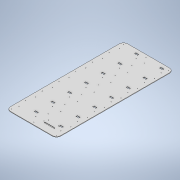
# Autodesk Inventor part: back_Box
Saved by Autodesk Inventor 2020 (Build 240168000, 168)
## iProperties
Created: 2020-07-08
Part Number: back_Box
Material: Generic
Document SubType Name: Modeling
Designer: gerac
Density: 1 g/cm^3
Appearance: Default
Author: gerac
Autodesk Inventor part; units mm, degrees
ref_plane "YZ Plane" through (0, 0, 0) normal (1, 0, 0) x (0, 1, 0)
ref_plane "XZ Plane" through (0, 0, 0) normal (0, 1, 0) x (-1, 0, 0)
ref_plane "XY Plane" through (0, 0, 0) normal (0, 0, 1) x (1, 0, 0)
sketch "Sketch1" plane through (0, 0, 0) normal (0, 1, 0) x (-1, 0, 0)
  line L0 (144, 336) -> (-144, 336)
  line L1 (-144, 336) -> (-144, -336)
  line L2 (-144, -336) -> (144, -336)
  line L3 (144, -336) -> (144, 336)
  line L4 (144, 336) -> (-144, -336) construction
  line L5 (-144, 336) -> (144, -336) construction
  circle A0 centre (-24, 288) radius 1.25
  circle A1 centre (-121, 288) radius 1.25
  circle A2 centre (-24, 192) radius 1.25
  circle A3 centre (-121, 192) radius 1.25
  circle A4 centre (-24, 96) radius 1.25
  circle A5 centre (-121, 96) radius 1.25
  circle A6 centre (-24, 0) radius 1.25
  circle A7 centre (-121, 0) radius 1.25
  circle A8 centre (-24, -96) radius 1.25
  circle A9 centre (-121, -96) radius 1.25
  circle A10 centre (-24, -192) radius 1.25
  circle A11 centre (-121, -192) radius 1.25
  circle A12 centre (-24, -288) radius 1.25
  circle A13 centre (-121, -288) radius 1.25
  circle A14 centre (120, 288) radius 1.25
  circle A15 centre (23, 288) radius 1.25
  circle A16 centre (120, 192) radius 1.25
  circle A17 centre (23, 192) radius 1.25
  circle A18 centre (120, 96) radius 1.25
  circle A19 centre (23, 96) radius 1.25
  circle A20 centre (120, 0) radius 1.25
  circle A21 centre (23, 0) radius 1.25
  circle A22 centre (120, -96) radius 1.25
  circle A23 centre (23, -96) radius 1.25
  circle A24 centre (120, -192) radius 1.25
  circle A25 centre (23, -192) radius 1.25
  circle A26 centre (120, -288) radius 1.25
  circle A27 centre (23, -288) radius 1.25
  line L6 (-92.1, 269) -> (-109.1, 269)
  line L7 (-109.1, 269) -> (-109.1, 261)
  line L8 (-109.1, 261) -> (-92.1, 261)
  line L9 (-92.1, 261) -> (-92.1, 269)
  line L10 (-92.1, 269) -> (-109.1, 261) construction
  line L11 (-109.1, 269) -> (-92.1, 261) construction
  line L12 (-92.1, 165) -> (-92.1, 173)
  line L13 (-92.1, 173) -> (-109.1, 173)
  line L14 (-109.1, 173) -> (-109.1, 165)
  line L15 (-109.1, 165) -> (-92.1, 165)
  line L16 (-92.1, 69) -> (-92.1, 77)
  line L17 (-92.1, 77) -> (-109.1, 77)
  line L18 (-109.1, 77) -> (-109.1, 69)
  line L19 (-109.1, 69) -> (-92.1, 69)
  line L20 (-92.1, -27) -> (-92.1, -19)
  line L21 (-92.1, -19) -> (-109.1, -19)
  line L22 (-109.1, -19) -> (-109.1, -27)
  line L23 (-109.1, -27) -> (-92.1, -27)
  line L24 (-92.1, -123) -> (-92.1, -115)
  line L25 (-92.1, -115) -> (-109.1, -115)
  line L26 (-109.1, -115) -> (-109.1, -123)
  line L27 (-109.1, -123) -> (-92.1, -123)
  line L28 (-92.1, -219) -> (-92.1, -211)
  line L29 (-92.1, -211) -> (-109.1, -211)
  line L30 (-109.1, -211) -> (-109.1, -219)
  line L31 (-109.1, -219) -> (-92.1, -219)
  line L32 (-92.1, -315) -> (-92.1, -307)
  line L33 (-92.1, -307) -> (-109.1, -307)
  line L34 (-109.1, -307) -> (-109.1, -315)
  line L35 (-109.1, -315) -> (-92.1, -315)
  line L36 (51.9, 261) -> (51.9, 269)
  line L37 (51.9, 269) -> (34.9, 269)
  line L38 (34.9, 269) -> (34.9, 261)
  line L39 (34.9, 261) -> (51.9, 261)
  line L40 (51.9, 165) -> (51.9, 173)
  line L41 (51.9, 173) -> (34.9, 173)
  line L42 (34.9, 173) -> (34.9, 165)
  line L43 (34.9, 165) -> (51.9, 165)
  line L44 (51.9, 69) -> (51.9, 77)
  line L45 (51.9, 77) -> (34.9, 77)
  line L46 (34.9, 77) -> (34.9, 69)
  line L47 (34.9, 69) -> (51.9, 69)
  line L48 (51.9, -27) -> (51.9, -19)
  line L49 (51.9, -19) -> (34.9, -19)
  line L50 (34.9, -19) -> (34.9, -27)
  line L51 (34.9, -27) -> (51.9, -27)
  line L52 (51.9, -123) -> (51.9, -115)
  line L53 (51.9, -115) -> (34.9, -115)
  line L54 (34.9, -115) -> (34.9, -123)
  line L55 (34.9, -123) -> (51.9, -123)
  line L56 (51.9, -219) -> (51.9, -211)
  line L57 (51.9, -211) -> (34.9, -211)
  line L58 (34.9, -211) -> (34.9, -219)
  line L59 (34.9, -219) -> (51.9, -219)
  line L60 (51.9, -315) -> (51.9, -307)
  line L61 (51.9, -307) -> (34.9, -307)
  line L62 (34.9, -307) -> (34.9, -315)
  line L63 (34.9, -315) -> (51.9, -315)
  point P0 (0, 0)
  point P1 (-100.6, 265)
  dimension "d0" = 288
  dimension "d1" = 672
  dimension "d4" = 2.5
  dimension "d5" = 2.5
  dimension "d6" = 97
  dimension "d7" = 23
  dimension "d8" = 48
  dimension "d9" = 48
  dimension "d12" = 96
  dimension "d15" = 144
  dimension "d20" = 17
  dimension "d21" = 8
  dimension "d22" = 71
  dimension "d23" = 43.4
  dimension "d26" = 96
  dimension "d29" = 144
  constraints: 128 end point, 28 centre point, 4 horizontal, 4 midpoint, 4 parallel, 2 perpendicular, 2 vertical, 156 other
  measures "d0" distance of L2.end L1.end
  measures "d1" distance of L1.end L0.end
  measures "d4" diameter of A1
  measures "d5" diameter of A0
  measures "d6" distance of A1.centre A0.centre
  measures "d7" distance from line of A1.centre L1
  measures "d8" distance from line of L0 A1.centre
  measures "d9" distance from line of L0 A0.centre
  measures "d12" distance of A0.centre A2.centre
  measures "d15" distance of A0.centre A14.centre
  measures "d20" distance between parallel lines of L7 L9
  measures "d21" distance between parallel lines of L6 L8
  measures "d22" distance from line of L0 point (-100.6, 265)
  measures "d23" distance from line of L1 point (-100.6, 265)
  measures "d26" distance of L8.end L12.start
  measures "d29" distance of L8.end L36.start
extrude "Extrusion3" add sketch "Sketch1" along normal blind 3
fillet "Fillet1" radius 24 4 edges at (-144, 1.5, 336) (-144, 1.5, -336) (144, 1.5, -336) (144, 1.5, 336)
sketch "Sketch2" plane through (0, 3, 0) normal (0, 1, 0) x (1, 0, 0)
  line L0 (28.5, -296.5) -> (93.5, -296.5)
  line L1 (93.5, -296.5) -> (93.5, -266.5)
  line L2 (93.5, -266.5) -> (28.5, -266.5)
  line L3 (28.5, -266.5) -> (28.5, -296.5)
  line L4 (28.5, -296.5) -> (93.5, -266.5) construction
  line L5 (93.5, -296.5) -> (28.5, -266.5) construction
  line L6 (144, -312) -> (144, 312) projected
  line L7 (-120, -336) -> (120, -336) projected
  line L8 (35, -296) -> (87, -296)
  line L9 (87, -296) -> (87, -290)
  line L10 (87, -290) -> (35, -290)
  line L11 (35, -290) -> (35, -296)
  line L12 (35, -296) -> (87, -290) construction
  line L13 (87, -296) -> (35, -290) construction
  circle A0 centre (32, -293) radius 1.375
  circle A1 centre (32, -270) radius 1.375
  circle A2 centre (90, -293) radius 1.375
  circle A3 centre (90, -270) radius 1.375
  point P0 (0, 0)
  point P1 (61, -281.5)
  point P2 (61, -293)
  dimension "d35" = 65
  dimension "d36" = 30
  dimension "d39" = 52
  dimension "d40" = 6
  dimension "d41" = 2.75
  dimension "d42" = 3.5
  dimension "d43" = 3.5
  dimension "d44" = 2.75
  dimension "d45" = 3.5
  dimension "d46" = 3.5
  dimension "d47" = 2.75
  dimension "d48" = 3.5
  dimension "d49" = 3.5
  dimension "d50" = 2.75
  dimension "d51" = 3.5
  dimension "d52" = 3.5
  dimension "d59" = 3.5
  dimension "d60" = 29
  dimension "d63" = 43
  dimension "d64" = 83
  constraints: 24 end point, 4 centre point, 4 midpoint, 4 parallel, 2 horizontal, 2 perpendicular
  measures "d35" distance of L2.end L1.end
  measures "d36" distance of L1.end L0.end
  measures "d39" distance of L10.end L9.end
  measures "d40" distance of L9.end L8.end
  measures "d41" diameter of A0
  measures "d42" distance from line of L3 A0.centre
  measures "d43" distance from line of L0 A0.centre
  measures "d44" diameter of A1
  measures "d45" distance from line of L2 A1.centre
  measures "d46" distance from line of L3 A1.centre
  measures "d47" diameter of A2
  measures "d48" distance from line of L1 A2.centre
  measures "d49" distance from line of L0 A2.centre
  measures "d50" diameter of A3
  measures "d51" distance from line of L2 A3.centre
  measures "d52" distance from line of L1 A3.centre
  measures "d59" distance from line of L0 point (61, -293)
  measures "d60" distance of A2.centre point (61, -293)
  measures "d63" distance from line of L7 point (61, -293)
  measures "d64" distance from line of L6 point (61, -293)
extrude "Extrusion4" cut sketch "Sketch2" against normal blind 1.5 contours L11 L10 L9 L8 | A0 | A1 | A2 | A3
sketch "Sketch6" plane through (0, 3, 0) normal (0, 1, 0) x (1, 0, 0)
  circle A0 centre (130, -322) radius 1.25
  line L0 (144, -312) -> (144, 312) projected
  line L1 (-120, -336) -> (120, -336) projected
  circle A1 centre (0, -322) radius 1.25
  circle A2 centre (-130, -322) radius 1.25
  circle A3 centre (130, 322) radius 1.25
  circle A4 centre (0, 322) radius 1.25
  circle A5 centre (-130, 322) radius 1.25
  circle A6 centre (130, -240) radius 1.25
  circle A7 centre (0, -240) radius 1.25
  circle A8 centre (-130, -240) radius 1.25
  circle A9 centre (130, -144) radius 1.25
  circle A10 centre (0, -144) radius 1.25
  circle A11 centre (-130, -144) radius 1.25
  circle A12 centre (130, -48) radius 1.25
  circle A13 centre (0, -48) radius 1.25
  circle A14 centre (-130, -48) radius 1.25
  circle A15 centre (130, 48) radius 1.25
  circle A16 centre (0, 48) radius 1.25
  circle A17 centre (-130, 48) radius 1.25
  circle A18 centre (130, 144) radius 1.25
  circle A19 centre (0, 144) radius 1.25
  circle A20 centre (-130, 144) radius 1.25
  circle A21 centre (130, 240) radius 1.25
  circle A22 centre (0, 240) radius 1.25
  circle A23 centre (-130, 240) radius 1.25
  point P0 (0, 0)
  dimension "d117" = 2.5
  dimension "d118" = 14
  dimension "d119" = 14
  dimension "d122" = 130
  dimension "d125" = 644
  dimension "d128" = 2.5
  dimension "d129" = 14
  dimension "d130" = 96
  dimension "d133" = 130
  dimension "d136" = 96
  constraints: 24 centre point, 2 horizontal, 2 vertical, 44 other
  measures "d117" diameter of A0
  measures "d118" distance from line of A0.centre L0
  measures "d119" distance from line of L1 A0.centre
  measures "d122" distance of A0.centre A1.centre
  measures "d125" distance of A0.centre A3.centre
  measures "d128" diameter of A6
  measures "d129" distance from line of L0 A6.centre
  measures "d130" distance from line of L1 A6.centre
  measures "d133" distance of A6.centre A7.centre
  measures "d136" distance of A6.centre A9.centre
extrude "Extrusion8" cut sketch "Sketch6" against normal blind 3
body "Solid3"
